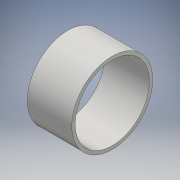
# Autodesk Inventor part: Bearing_Silicone
Saved by Autodesk Inventor 2016 (Build 200138000, 138)
## iProperties
Created: 2016-01-06
Part Number: Bearing_Silicone
Material: UHMW, White
Document SubType Name: Modeling
Designer: m2memari
Density: 0.94 g/cm^3
Appearance: Smooth - White
Author: m2memari
Autodesk Inventor part; units mm, degrees
ref_plane "YZ Plane" through (0, 0, 0) normal (1, 0, 0) x (0, 1, 0)
ref_plane "XZ Plane" through (0, 0, 0) normal (0, 1, 0) x (-1, 0, 0)
ref_plane "XY Plane" through (0, 0, 0) normal (0, 0, 1) x (1, 0, 0)
sketch "Sketch1" plane through (0, 0, 0) normal (1, 0, 0) x (0, 1, 0)
  circle A0 centre (0, 0) radius 12
  circle A1 centre (0, 0) radius 11
  dimension "d0" = 24
  dimension "d1" = 22
  constraints: 2 centre point, 2 coincident
  measures "d0" diameter of A0
  measures "d1" diameter of A1
extrude "Extrusion1" add sketch "Sketch1" along normal mid plane 13.2
equation "\"d0\" = BearingDiameter"
equation "\"d2\" = BearingSiliconeWidth"
equation "\"BearingDiameter\" = 24"
equation "\"BearingSiliconeWidth\" = 13.2"
body "Solid1"
